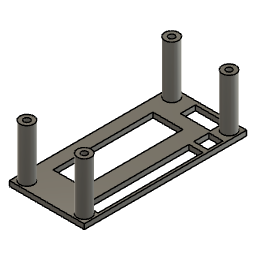
rpi_holder (Autodesk Fusion 360 design; units mm, degrees)
Autodesk Fusion 360 part; units mm, degrees
sketch "Sketch1" plane through (0, 0, 0) normal (0, 1, 0) x (1, 0, 0)
  line L0 (15, 32.5) -> (-15, 32.5)
  line L1 (-15, 32.5) -> (-15, -32.5)
  line L2 (-15, -32.5) -> (15, -32.5)
  line L3 (15, -32.5) -> (15, 32.5)
  line L4 (15, 32.5) -> (-15, -32.5) construction
  line L5 (-15, 32.5) -> (15, -32.5) construction
  dimension "d1" = 30
  dimension "d2" = 65
  constraint horizontal L0
  constraint perpendicular L0 L1
  constraint parallel L0 L2
  constraint parallel L1 L3
  constraint coincident L4 origin
  constraint coincident L5 origin
  measures "d1" distance of L1.end L2.end
  measures "d2" distance of L0.end L1.end
extrude "Extrude1" add sketch "Sketch1" along normal blind 2
sketch "Sketch2" plane through (0, 2, 0) normal (0, 1, 0) x (-1, 0, 0)
  line L0 (-15, 32.5) -> (-15, -32.5)
  line L1 (-15, -32.5) -> (15, -32.5)
  line L2 (15, -32.5) -> (15, 32.5)
  line L3 (15, 32.5) -> (-15, 32.5)
  circle A0 centre (-11.5, -29) radius 2.8
  circle A1 centre (11.5, -29) radius 2.8
  circle A2 centre (-11.5, 29) radius 2.8
  circle A3 centre (11.5, 29) radius 2.8
  dimension "d5" = 5.6
  dimension "d6" = 3.5
  dimension "d7" = 3.5
  dimension "d8" = 5.6
  dimension "d9" = 3.5
  dimension "d10" = 3.5
  dimension "d11" = 5.6
  dimension "d12" = 3.5
  dimension "d13" = 3.5
  dimension "d14" = 5.6
  dimension "d15" = 3.5
  dimension "d16" = 3.5
  measures "d5" diameter of A0
  measures "d6" distance of L0 A0.centre
  measures "d7" distance of L1 A0.centre
  measures "d8" diameter of A1
  measures "d9" distance of L1 A1.centre
  measures "d10" distance of L2 A1.centre
  measures "d11" diameter of A2
  measures "d12" distance of L3 A2.centre
  measures "d13" distance of L0 A2.centre
  measures "d14" diameter of A3
  measures "d15" distance of L3 A3.centre
  measures "d16" distance of L2 A3.centre
extrude "Extrude2" add sketch "Sketch2" along normal blind 21 contours A0 | A1 | A2 | A3
sketch "Sketch3" plane through (0, 23, 0) normal (0, 1, 0) x (-1, 0, 0)
  circle A0 centre (-11.5, -29) radius 2.8
  circle A1 centre (-11.5, -29) radius 1.2
  circle A2 centre (11.5, -29) radius 1.2
  circle A3 centre (11.5, -29) radius 2.8
  circle A4 centre (-11.5, 29) radius 1.2
  circle A5 centre (-11.5, 29) radius 2.8
  circle A6 centre (11.5, 29) radius 1.2
  circle A7 centre (11.5, 29) radius 2.8
  dimension "d19" = 2.4
  dimension "d20" = 2.4
  dimension "d21" = 2.4
  dimension "d22" = 2.4
  constraint concentric A0 A1
  constraint concentric A2 A3
  constraint concentric A4 A5
  constraint concentric A6 A7
  measures "d19" diameter of A1
  measures "d20" diameter of A2
  measures "d21" diameter of A4
  measures "d22" diameter of A6
extrude "Extrude3" cut sketch "Sketch3" against normal blind 5 contours A1 | A2 | A4 | A6
sketch "Sketch4" plane through (0, 2, 0) normal (0, 1, 0) x (-1, 0, 0)
  circle A0 centre (11.5, -29) radius 2.8
  circle A1 centre (11.5, 29) radius 2.8
  circle A2 centre (-11.5, -29) radius 2.8
  circle A3 centre (-11.5, 29) radius 2.8
  line L0 (-15, 32.5) -> (-15, -32.5)
  line L1 (-15, -32.5) -> (15, -32.5)
  line L2 (15, -32.5) -> (15, 32.5)
  line L3 (15, 32.5) -> (-15, 32.5)
  line L4 (-14, 26) -> (-8.4, 26)
  line L5 (-8.4, 26) -> (-8.4, -24)
  line L6 (-8.4, -24) -> (-14, -24)
  line L7 (-14, -24) -> (-14, 26)
  dimension "d25" = 5.6
  dimension "d26" = 6.5
  dimension "d27" = 1
  dimension "d28" = 50
  constraint horizontal L4
  constraint vertical L5
  constraint horizontal L6
  constraint vertical L7
  measures "d25" distance of L4.start L4.end
  measures "d26" distance of L3 L4
  measures "d27" distance of L0 L7
  measures "d28" distance of L4.end L5.end
extrude "Extrude4" cut sketch "Sketch4" against normal blind 5 contours L4 L5 L6 L7
sketch "Sketch5" plane through (0, 2, 0) normal (0, 1, 0) x (-1, 0, 0)
  line L0 (-8.4, 26) -> (-8.4, -24)
  line L1 (-8.4, -24) -> (-14, -24)
  line L2 (-14, -24) -> (-14, 26)
  line L3 (-14, 26) -> (-8.4, 26)
  circle A0 centre (11.5, -29) radius 2.8
  circle A1 centre (11.5, 29) radius 2.8
  circle A2 centre (-11.5, -29) radius 2.8
  circle A3 centre (-11.5, 29) radius 2.8
  line L4 (-15, 32.5) -> (-15, -32.5)
  line L5 (-15, -32.5) -> (15, -32.5)
  line L6 (15, -32.5) -> (15, 32.5)
  line L7 (15, 32.5) -> (-15, 32.5)
  line L8 (-14, -18) -> (-8, -18)
  line L9 (-8, -18) -> (-8, -16)
  line L10 (-8, -16) -> (-14, -16)
  line L11 (-14, -16) -> (-14, -18)
  dimension "d31" = 6
  dimension "d32" = 2
  constraint horizontal L8
  constraint vertical L9
  constraint horizontal L10
  constraint vertical L11
  constraint coincident L2 L8.start
  measures "d31" distance of L8.start L8.end
  measures "d32" distance of L8.start L10.end
extrude "Extrude5" add sketch "Sketch5" against normal blind 2 contours L0 L2 L8 L10 L11
sketch "Sketch6" plane through (0, 2, 0) normal (0, 1, 0) x (-1, 0, 0)
  line L0 (-14, -16) -> (-14, 26)
  line L1 (-14, 26) -> (-8.4, 26)
  line L2 (-8.4, 26) -> (-8.4, -16)
  line L3 (-8.4, -16) -> (-14, -16)
  line L4 (-14, -18) -> (-8.4, -18)
  line L5 (-8.4, -18) -> (-8.4, -24)
  line L6 (-8.4, -24) -> (-14, -24)
  line L7 (-14, -24) -> (-14, -18)
  circle A0 centre (11.5, -29) radius 2.8
  circle A1 centre (11.5, 29) radius 2.8
  circle A2 centre (-11.5, -29) radius 2.8
  circle A3 centre (-11.5, 29) radius 2.8
  line L8 (-15, 32.5) -> (-15, -32.5)
  line L9 (-15, -32.5) -> (15, -32.5)
  line L10 (15, -32.5) -> (15, 32.5)
  line L11 (15, 32.5) -> (-15, 32.5)
  line L12 (10, 20) -> (-2, 20)
  line L13 (-2, 20) -> (-2, -20)
  line L14 (-2, -20) -> (10, -20)
  line L15 (10, -20) -> (10, 20)
  constraint horizontal L12
  constraint vertical L13
  constraint horizontal L14
  constraint vertical L15
extrude "Extrude6" cut sketch "Sketch6" against normal blind 2 contours L12 L13 L14 L15
sketch "Sketch7" plane through (0, 2, 0) normal (0, 1, 0) x (-1, 0, 0)
  line L0 (-2, 20) -> (10, 20)
  line L1 (10, 20) -> (10, -20)
  line L2 (10, -20) -> (-2, -20)
  line L3 (-2, -20) -> (-2, 20)
  line L4 (-14, -16) -> (-14, 26)
  line L5 (-14, 26) -> (-8.4, 26)
  line L6 (-8.4, 26) -> (-8.4, -16)
  line L7 (-8.4, -16) -> (-14, -16)
  line L8 (-14, -18) -> (-8.4, -18)
  line L9 (-8.4, -18) -> (-8.4, -24)
  line L10 (-8.4, -24) -> (-14, -24)
  line L11 (-14, -24) -> (-14, -18)
  circle A0 centre (11.5, -29) radius 2.8
  circle A1 centre (11.5, 29) radius 2.8
  circle A2 centre (-11.5, -29) radius 2.8
  circle A3 centre (-11.5, 29) radius 2.8
  line L12 (-15, 32.5) -> (-15, -32.5)
  line L13 (-15, -32.5) -> (15, -32.5)
  line L14 (15, -32.5) -> (15, 32.5)
  line L15 (15, 32.5) -> (-15, 32.5)
  line L16 (-8, -31) -> (4, -31)
  line L17 (4, -31) -> (4, -25)
  line L18 (4, -25) -> (-8, -25)
  line L19 (-8, -25) -> (-8, -31)
  constraint horizontal L16
  constraint vertical L17
  constraint horizontal L18
  constraint vertical L19
extrude "Extrude7" cut sketch "Sketch7" against normal blind 2 contours L16 L17 L18 L19
